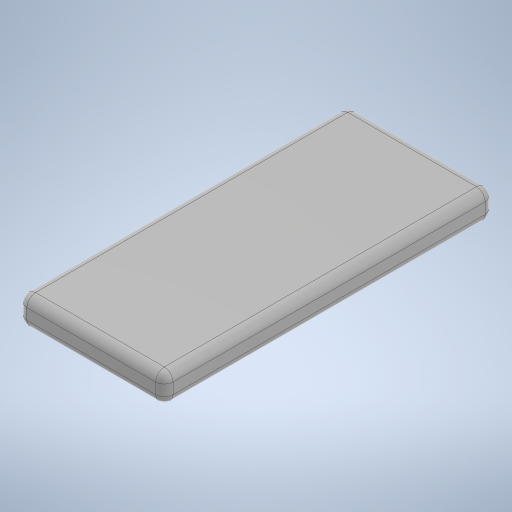
# Autodesk Inventor part: Matress
Saved by Autodesk Inventor 2023 (Build 270158000, 158)
## iProperties
Created: 2022-10-13
Part Number: Matress
Material: Rubber
Document SubType Name: Modeling
Designer: mliu-23
Density: 0.93 g/cm^3
Appearance: Smooth - Medium Gray
Author: mliu-23
Autodesk Inventor part; units mm, degrees
ref_plane "YZ Plane" through (0, 0, 0) normal (1, 0, 0) x (0, 1, 0)
ref_plane "XZ Plane" through (0, 0, 0) normal (0, 1, 0) x (-1, 0, 0)
ref_plane "XY Plane" through (0, 0, 0) normal (0, 0, 1) x (1, 0, 0)
sketch "Sketch1" plane through (0, 0, 0) normal (0, 1, 0) x (-1, 0, 0)
  line L0 (-425.45, 958.85) -> (425.45, 958.85)
  line L1 (425.45, 958.85) -> (425.45, -958.85)
  line L2 (425.45, -958.85) -> (-425.45, -958.85)
  line L3 (-425.45, -958.85) -> (-425.45, 958.85)
  line L4 (-425.45, 958.85) -> (425.45, -958.85) construction
  line L5 (425.45, 958.85) -> (-425.45, -958.85) construction
  point P0 (0, 0)
  dimension "d0" = 850.9
  dimension "d1" = 1917.7
  constraints: 12 end point, 2 midpoint, 2 parallel, 1 horizontal, 1 perpendicular
  measures "d0" distance of L1.end L2.end
  measures "d1" distance of L0.end L1.end
extrude "Extrusion1" add sketch "Sketch1" along normal blind 165.1
fillet "Fillet1" radius 50.8 12 edges at (425.45, 165.1, 0) (-425.45, 165.1, 0) (425.45, 0, 0) (-425.45, 0, 0) (0, 165.1, 958.85) (0, 0, 958.85) (425.45, 82.55, 958.85) (-425.45, 82.55, 958.85) (425.45, 82.55, -958.85) (0, 165.1, -958.85) (0, 0, -958.85) (-425.45, 82.55, -958.85)
body "Solid1"
